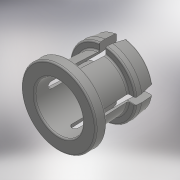
# Autodesk Inventor part: Clip pneumatique
Saved by Autodesk Inventor 2017 (Build 210142000, 142)
## iProperties
Company: FABLAB Frenchmakers
Part Number: Clip pneumatique
Material: Plastique ABS
Document SubType Name: Modeling
Designer: FABLAB Frenchmakers
Density: 1.06 g/cm^3
Appearance: Lisse - Blanc(1)
Mass: 0.169604 g
Surface Area: 4.93315 cm^2
Volume: 0.160003 cm^3
Project: 1420 Vauban 3D XL
Catalog Web Link: http://frenchmakers.com/
Stock Number: 1420-02-26
Autodesk Inventor part; units mm, degrees
ref_plane "YZ Plane" through (0, 0, 0) normal (1, 0, 0) x (0, 1, 0)
ref_plane "XZ Plane" through (0, 0, 0) normal (0, 1, 0) x (-1, 0, 0)
ref_plane "XY Plane" through (0, 0, 0) normal (0, 0, 1) x (1, 0, 0)
sketch "Esquisse1" plane through (0, 0, 0) normal (0, 0, 1) x (1, 0, 0)
  line L0 (0, 0) -> (5.075, 0)
  line L1 (5.075, 0) -> (5.075, 1.5)
  line L2 (5.075, 1.5) -> (3.725, 1.5)
  line L3 (3.725, 1.5) -> (3.5, 6)
  line L4 (3.5, 6) -> (4.5, 6)
  line L5 (4.5, 6) -> (4.5, 6.85)
  line L6 (4.5, 6.85) -> (4.25, 8.6)
  line L7 (4.25, 8.6) -> (0, 8.6)
  line L8 (0, 8.6) -> (0, 0)
  line L9 (0, 0) -> (0, 11.7685)
  dimension "d1" = 10.15
  dimension "d2" = 8.6
  dimension "d3" = 1.5
  dimension "d4" = 4.5
  dimension "d5" = 7.45
  dimension "d6" = 7
  dimension "d7" = 9
  dimension "d8" = 8.5
  dimension "d9" = 0.85
  constraints: 20 end point, 4 perpendicular, 2 parallel, 1 horizontal, 1 vertical
  measures "d1" diameter of L1 L9
  measures "d2" distance between parallel lines of L0 L7
  measures "d3" distance between parallel lines of L0 L2
  measures "d4" distance between parallel lines of L2 L4
  measures "d5" diameter of L2.end L9
  measures "d6" diameter of L3.end L9
  measures "d7" diameter of L5 L9
  measures "d8" diameter of L6.end L9
  measures "d9" distance of L4.end L5.end
revolve "Révolution1" add sketch "Esquisse1" angle 360 about axis through (0, 0, 0) along (0, 1, 0)
sketch "Esquisse2" plane through (0, 0, 0) normal (0, -1, 0) x (1, 0, 0)
  point P0 (0, 0)
  point P1 (0, 0)
  constraints: 1 coincident
hole "Perçage1" at (0, 0, 0) direction (0, 1, 0) diameter 6.5 end through all
fillet "Congé1" radius 0.2 7 edges at (-4.25, 8.6, 0) (0, 8.6, 3.25) (-5.075, 1.5, 0) (-5.075, 0, 0) (0, 0, 3.25) (-4.5, 6, 0) (-3.5, 6, 0)
sketch "Esquisse3" plane through (0, 0, 0) normal (1, 0, 0) x (0, 1, 0)
  line L0 (8.6, 0.7) -> (6.1, 0.45)
  line L1 (6.1, 0.45) -> (2.3, 0.45)
  arc A0 (2.3, 0.45) -> (2.3, -0.45) centre (2.3, 0) ccw
  line L2 (2.3, -0.45) -> (6.1, -0.45)
  line L3 (6.1, -0.45) -> (8.6, -0.7)
  line L4 (8.6, -0.7) -> (8.6, 0.7)
  line L5 (8.6, 3.25) -> (8.6, -3.25) construction
  point P0 (0, 0)
  point P1 (8.6, 0)
  dimension "d18" = 0.9
  dimension "d19" = 6.3
  dimension "d20" = 1.4
  dimension "d21" = 2.5
  constraints: 10 end point, 2 point on circle, 2 tangent, 1 centre point, 1 collinear, 1 equal length, 1 horizontal alignment, 1 midpoint, 1 parallel, 1 perpendicular, 1 vertical alignment
  measures "d18" diameter of A0
  measures "d19" distance from line of L5 A0.centre
  measures "d20" distance of L3.end L0.start
  measures "d21" distance from line of L5 L0.end
extrude "Extrusion1" cut sketch "Esquisse3" along normal through all both and the other way through all
pattern_circular "Réseau circulaire1" count 2 over 90 about axis through (0, 16.7333, 0) along (0, -1, 0) of "Extrusion1"
